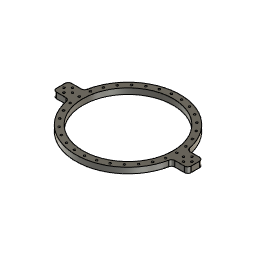
flange v2 (Autodesk Fusion 360 design; units mm, degrees)
Autodesk Fusion 360 part; units mm, degrees
sketch "Sketch1" plane through (0, 0, 0) normal (0, 0, 1) x (1, 0, 0)
  arc A0 (-114.2774, -23.019) -> (114.2774, -23.019) centre (0, 0) ccw
  circle A1 centre (-73.0021, 81.0771) radius 2.1527
  circle A2 centre (-88.2638, -64.1274) radius 2.1527
  circle A3 centre (73.0021, -81.0771) radius 2.1527
  circle A4 centre (-143.1, 0) radius 2.1525
  arc A5 (-114.2774, -23.019) -> (-121.6297, -17) centre (-121.6297, -24.5) ccw
  circle A6 centre (11.4041, 108.5023) radius 2.1526
  circle A7 centre (-54.55, -94.4834) radius 2.1527
  circle A8 centre (-109.1, 0) radius 2.1527
  circle A9 centre (88.2638, 64.1274) radius 2.1527
  circle A10 centre (143.1, 0) radius 2.1525
  circle A11 centre (54.55, 94.4834) radius 2.1527
  circle A12 centre (54.55, -94.4834) radius 2.1527
  circle A13 centre (106.7159, 22.6832) radius 2.1527
  circle A14 centre (133.6, -9.5) radius 2.1525
  circle A15 centre (-33.7138, 103.7603) radius 2.1526
  circle A16 centre (124.1, 0) radius 2.1525
  line L0 (143.1, 17) -> (121.6297, 17)
  circle A17 centre (109.1, 0) radius 2.1526
  circle A18 centre (-133.6, -9.5) radius 2.1525
  circle A19 centre (-99.6678, 44.375) radius 2.1527
  circle A20 centre (-133.6, 9.5) radius 2.1525
  line L1 (-121.6297, 17) -> (-143.1, 17)
  circle A21 centre (11.4041, -108.5023) radius 2.1526
  line L2 (150.6, -9.5) -> (150.6, 9.5)
  circle A22 centre (-88.2638, 64.1274) radius 2.1527
  circle A23 centre (133.6, 9.5) radius 2.1525
  line L3 (-150.6, 9.5) -> (-150.6, -9.5)
  line L4 (121.6297, -17) -> (143.1, -17)
  circle A24 centre (33.7138, -103.7603) radius 2.1526
  circle A25 centre (0, 0) radius 100.965
  arc A26 (114.2774, 23.019) -> (121.6297, 17) centre (121.6297, 24.5) ccw
  circle A27 centre (-124.1, 0) radius 2.1525
  line L5 (-143.1, -17) -> (-121.6297, -17)
  circle A28 centre (73.0021, 81.0771) radius 2.1527
  circle A29 centre (-33.7138, -103.7603) radius 2.1527
  arc A30 (150.6, 9.5) -> (143.1, 17) centre (143.1, 9.5) ccw
  circle A31 centre (-99.6678, -44.375) radius 2.1527
  arc A32 (121.6297, -17) -> (114.2774, -23.019) centre (121.6297, -24.5) ccw
  circle A33 centre (88.2638, -64.1274) radius 2.1527
  arc A34 (-143.1, 17) -> (-150.6, 9.5) centre (-143.1, 9.5) ccw
  circle A35 centre (-11.4041, 108.5023) radius 2.1526
  circle A36 centre (99.6678, 44.375) radius 2.1527
  circle A37 centre (99.6678, -44.375) radius 2.1527
  circle A38 centre (-54.55, 94.4834) radius 2.1527
  circle A39 centre (33.7138, 103.7603) radius 2.1527
  arc A40 (114.2774, 23.019) -> (-114.2774, 23.019) centre (0, 0) ccw
  circle A41 centre (-106.7159, 22.6832) radius 2.1527
  arc A42 (143.1, -17) -> (150.6, -9.5) centre (143.1, -9.5) ccw
  circle A43 centre (106.7159, -22.6832) radius 2.1526
  circle A44 centre (-106.7159, -22.6832) radius 2.1527
  arc A45 (-121.6297, 17) -> (-114.2774, 23.019) centre (-121.6297, 24.5) ccw
  arc A46 (-150.6, -9.5) -> (-143.1, -17) centre (-143.1, -9.5) ccw
  circle A47 centre (-11.4041, -108.5023) radius 2.1526
  circle A48 centre (-73.0021, -81.0771) radius 2.1527
extrude "Extrude1" add sketch "Sketch1" along normal blind 12.7
